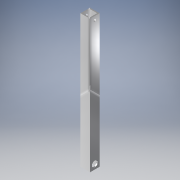
# Autodesk Inventor part: 15102898-16-A-0301
Saved by Autodesk Inventor 2017 (Build 210142000, 142)
## iProperties
Created: 2016-10-02
Part Number: 15102898-16-A-0301
Material: Aluminum 6061
Document SubType Name: Modeling
Designer: gus
Density: 2.7 g/cm^3
Appearance: Aluminum - Flat
Author: gus
Autodesk Inventor part; units mm, degrees
ref_plane "YZ Plane" through (0, 0, 0) normal (1, 0, 0) x (0, 1, 0)
ref_plane "XZ Plane" through (0, 0, 0) normal (0, 1, 0) x (-1, 0, 0)
ref_plane "XY Plane" through (0, 0, 0) normal (0, 0, 1) x (1, 0, 0)
sketch "Sketch1" plane through (0, 0, 0) normal (0, 1, 0) x (-1, 0, 0)
  line L0 (0, 0) -> (-25.4, 0)
  line L1 (-25.4, 0) -> (-25.4, 25.4)
  line L2 (-25.4, 25.4) -> (0, 25.4)
  line L3 (0, 25.4) -> (0, 0)
  line L4 (-3.175, 3.175) -> (-22.225, 3.175)
  line L5 (-22.225, 3.175) -> (-22.225, 22.225)
  line L6 (-22.225, 22.225) -> (-3.175, 22.225)
  line L7 (-3.175, 22.225) -> (-3.175, 3.175)
  dimension "d0" = 25.4
  dimension "d1" = 25.4
  dimension "d2" = 3.175
  constraints: 16 end point, 4 parallel, 2 perpendicular, 1 horizontal, 3 other
  measures "d0" distance of L1.end L2.end
  measures "d1" distance of L0.end L1.end
  measures "d2" distance between parallel lines of L3 L7
extrude "Extrusion1" add sketch "Sketch1" along normal blind 355.6
sketch "Sketch2" plane through (25.4, 0, 25.4) normal (1, 0, 0) x (0, 0, -1)
  circle A0 centre (12.7, 12.7) radius 7.9375
  line L0 (25.4, 0) -> (25.4, 355.6) projected
  line L1 (25.4, 0) -> (0, 0) projected
  dimension "d5" = 15.875
  dimension "d6" = 12.7
  dimension "d7" = 12.7
  constraints: 1 centre point
  measures "d5" diameter of A0
  measures "d6" distance from line of L0 A0.centre
  measures "d7" distance from line of L1 A0.centre
extrude "Extrusion2" cut sketch "Sketch2" against normal blind 25.4
sketch "Sketch3" plane through (0, 0, 0) normal (-1, 0, 0) x (0, 0, 1)
  line L0 (25.4, 0) -> (25.4, 355.6) projected
  line L1 (0, 355.6) -> (25.4, 355.6) projected
  point P0 (0, 0)
  point P1 (12.7, 346.075)
  dimension "d10" = 12.7
  dimension "d11" = 9.525
  measures "d10" distance from line of L0 point (12.7, 346.075)
  measures "d11" distance from line of L1 point (12.7, 346.075)
hole "Hole1" at (0, 346.075, 12.7) direction (1, 0, 0) diameter 6.35 end through all
body "Solid1"
